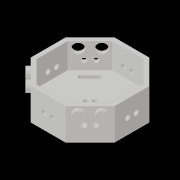
# Autodesk Inventor part: oktagonOben_v2
Saved by Autodesk Inventor 2018.2 (Build 222227000, 227)
## iProperties
Created: 2018-08-16
Part Number: oktagonOben_v2
Material: Generisch
Document SubType Name: Modeling
Designer: PRYADUN
Density: 1 g/cm^3
Appearance: Vorgabe
Mass: 6.7855 g
Surface Area: 62.9444 cm^2
Volume: 6.7855 cm^3
Author: PRYADUN
Autodesk Inventor part; units mm, degrees
sketch "Skizze1" plane through (0, 0, 0) normal (0, 0, 1) x (1, 0, 0)
  line L0 (-8.2843, 20) -> (8.2843, 20)
  line L1 (8.2843, 20) -> (20, 8.2843)
  line L2 (20, 8.2843) -> (20, -8.2843)
  line L3 (20, -8.2843) -> (8.2843, -20)
  line L4 (8.2843, -20) -> (-8.2843, -20)
  line L5 (-8.2843, -20) -> (-20, -8.2843)
  line L6 (-20, -8.2843) -> (-20, 8.2843)
  line L7 (-20, 8.2843) -> (-8.2843, 20)
  line L8 (0, -28) -> (0, 28) projected
  line L9 (-28, 0) -> (28, 0) projected
  point P0 (0, 0)
  dimension "d0" = 40
  dimension "d1" = 40
  constraints: 16 end point, 2 equal length, 2 horizontal, 1 perpendicular, 1 vertical, 5 other
  measures "d0" distance between parallel lines of L4 L0
  measures "d1" distance between parallel lines of L2 L6
extrude "Extrusion1" add sketch "Skizze1" along normal blind 15
sketch "Skizze2" plane through (0, 0, 15) normal (0, 0, 1) x (1, 0, 0)
  line L0 (8.2843, 20) -> (-8.2843, 20) projected
  line L1 (-8.2843, 20) -> (-20, 8.2843) projected
  line L2 (-20, 8.2843) -> (-20, -8.2843) projected
  line L3 (-20, -8.2843) -> (-8.2843, -20) projected
  line L4 (-8.2843, -20) -> (8.2843, -20) projected
  line L5 (8.2843, -20) -> (20, -8.2843) projected
  line L6 (20, -8.2843) -> (20, 8.2843) projected
  line L7 (20, 8.2843) -> (8.2843, 20) projected
  line L8 (-7.4558, 18) -> (7.4558, 18)
  line L9 (7.4558, 18) -> (18, 7.4558)
  line L10 (18, 7.4558) -> (18, -7.4558)
  line L11 (18, -7.4558) -> (7.4558, -18)
  line L12 (7.4558, -18) -> (-7.4558, -18)
  line L13 (-7.4558, -18) -> (-18, -7.4558)
  line L14 (-18, -7.4558) -> (-18, 7.4558)
  line L15 (-18, 7.4558) -> (-7.4558, 18)
  point P0 (0, 0)
  dimension "d4" = 2
  constraints: 16 end point, 7 other
  measures "d4" distance between parallel lines of L0 L8
extrude "Extrusion2" cut sketch "Skizze2" against normal blind 12 contours L8 L9 L10 L11 L12 L13 L14 L15
sketch "Skizze3" plane through (-18, -7.4558, 15) normal (1, 0, 0) x (0, 0, -1)
  line L0 (0, 0) -> (0, 14.9117) projected
  line L1 (0, 0) -> (12, 0) projected
  line L2 (12, 0) -> (12, 14.9117) projected
  line L3 (0, 14.9117) -> (12, 14.9117) projected
  line L4 (12, 0) -> (12, 14.9117) projected
  line L5 (12, 7.4558) -> (0, 7.4558)
  line L6 (0, 0) -> (0, 14.9117) projected
  point P0 (15, 7.4558)
  point P1 (8, 9.4558)
  point P2 (8, 5.4558)
  dimension "d7" = 4
  dimension "d23" = 4
  constraints: 2 end point, 2 midpoint, 1 symmetric about line, 1 vertical alignment
  measures "d7" distance of point (8, 5.456) point (8, 9.456)
  measures "d23" distance from line of L2 point (8, 9.456)
hole "Bohrung1" at (-18, 2, 7) at (-18, -2, 7) direction (-1, 0, 0) diameter 2.2 end through all
mirror "Spiegeln1" about plane through (0, 0, 0) normal (1, 0, 0) of "Bohrung1"
ref_plane "Arbeitsebene1" through (-5.2721, -5.2721, 15) normal (0.7071, -0.7071, 0) x (-0.7071, -0.7071, 0)
mirror "Spiegeln2" about plane through (-5.2721, -5.2721, 15) normal (0.7071, -0.7071, 0) of "Bohrung1"
sketch "Skizze4" plane through (-7.4558, -18, 3) normal (0.7071, 0.7071, 0) x (-0.7071, 0.7071, 0)
  point P0 (7.4558, -3)
ref_plane "Arbeitsebene2" through (-18, -7.4558, 15) normal (0.3827, -0.9239, 0) x (0, 0, -1)
mirror "Spiegeln3" about plane through (-18, -7.4558, 15) normal (0.3827, -0.9239, 0) of "Bohrung1"
mirror "Spiegeln4" about plane through (0, 0, 0) normal (0, 1, 0) of "Bohrung1", "Spiegeln2"
mirror "Spiegeln5" about plane through (0, 0, 0) normal (1, 0, 0) of "Bohrung1", "Spiegeln3"
mirror "Spiegeln6" about plane through (0, 0, 0) normal (0, 1, 0) of "Bohrung1", "Spiegeln3", "Spiegeln5"
sketch "Skizze6" plane through (-8.2843, -20, 15) normal (-0.7071, -0.7071, 0) x (-0.7071, 0.7071, 0)
  circle A0 centre (4.2843, 3.0841) radius 2.3005
  circle A1 centre (6.2843, 8) radius 1.1 projected
  circle A2 centre (10.2843, 8) radius 1.1 projected
  line L0 (0, 15) -> (16.5685, 15) projected
  line L1 (0, 15) -> (0, 0) projected
  line L2 (16.5685, 0) -> (0, 0) projected
  line L3 (16.5685, 15) -> (16.5685, 0) projected
  circle A3 centre (12.2843, 3.0841) radius 2.3005
  line L4 (8.2843, 15) -> (8.2843, 0)
  line L5 (16.5685, 0) -> (0, 0) projected
  dimension "d24" = 4.601
  dimension "d25" = 4.601
  dimension "d26" = 8
  constraints: 2 centre point, 2 end point, 1 horizontal alignment, 1 midpoint, 1 symmetric about line
  measures "d24" diameter of A0
  measures "d25" diameter of A3
  measures "d26" distance of A3.centre A0.centre
extrude "Extrusion3" add sketch "Skizze6" along normal blind 1.8 contours A0 | A3
chamfer "Fase1" distance 0.135 angle 45 2 edges at (-10.9598, -19.8701, 11.9159) (-16.6167, -14.2132, 11.9159)
sketch "Skizze7" plane through (8.2843, 20, 0) normal (0.7071, 0.7071, 0) x (-0.7071, 0.7071, 0)
  circle A0 centre (-4.2843, 11.9159) radius 2.3005 projected
  circle A1 centre (-12.2843, 11.9159) radius 2.3005 projected
  circle A2 centre (-4.2843, 11.9159) radius 2.3985
  circle A3 centre (-12.2843, 11.9159) radius 2.3985
  point P0 (-8.2843, 0)
  dimension "d33" = 4.797
  dimension "d34" = 4.797
  constraints: 2 centre point, 2 coincident
  measures "d33" diameter of A2
  measures "d34" diameter of A3
extrude "Extrusion4" cut sketch "Skizze7" against normal blind 2.2 contours A0 | A1 | A2 | A3
sketch "Skizze8" plane through (0, 0, 0) normal (0, 0, -1) x (-1, 0, 0)
  line L0 (8.2843, 20) -> (-8.2843, 20) projected
  line L1 (-8.2843, 20) -> (-20, 8.2843) projected
  line L2 (-20, 8.2843) -> (-20, -8.2843) projected
  line L3 (-20, -8.2843) -> (-8.2843, -20) projected
  line L4 (-8.2843, -20) -> (8.2843, -20) projected
  line L5 (8.2843, -20) -> (20, -8.2843) projected
  line L6 (20, -8.2843) -> (20, 8.2843) projected
  line L7 (20, 8.2843) -> (8.2843, 20) projected
  line L8 (8.2843, -20) -> (20, -8.2843) projected
  line L9 (14.1421, -14.1421) -> (-14.1421, 14.1421)
  line L10 (-20, 8.2843) -> (-8.2843, 20) projected
  point P0 (0, 0)
  point P1 (1.0607, -1.0607)
  point P2 (-1.0607, 1.0607)
  dimension "d43" = 3
  dimension "d44" = 1.5
  constraints: 2 end point, 2 midpoint, 2 point on line
  measures "d43" distance of point (-1.061, 1.061) point (1.061, -1.061)
  measures "d44" distance of point (0, 0) point (1.061, -1.061)
hole "Bohrung3" at (-1.0607, -1.0607, 0) at (1.0607, 1.0607, 0) direction (0, 0, 1) diameter 1.8 end through all
ref_plane "Arbeitsebene3" through (0, -18, 15) normal (1, 0, 0) x (0, 1, 0)
mirror "Spiegeln7" about plane through (0, -18, 15) normal (1, 0, 0) of "Extrusion3", "Extrusion4"
sketch "Skizze9" plane through (0, 0, 0) normal (0, 0, -1) x (-1, 0, 0)
  circle A0 centre (1.0607, -1.0607) radius 0.9 projected
  circle A1 centre (-1.0607, 1.0607) radius 0.9 projected
  line L0 (8.2843, 20) -> (-8.2843, 20) projected
  line L1 (-8.2843, 20) -> (-20, 8.2843) projected
  line L2 (-20, 8.2843) -> (-20, -8.2843) projected
  line L3 (-20, -8.2843) -> (-8.2843, -20) projected
  line L4 (-8.2843, -20) -> (8.2843, -20) projected
  line L5 (8.2843, -20) -> (20, -8.2843) projected
  line L6 (20, -8.2843) -> (20, 8.2843) projected
  line L7 (20, 8.2843) -> (8.2843, 20) projected
  line L8 (7.0004, 12.7986) -> (7.0004, 12.7986)
  line L9 (7.0004, 11.243) -> (11.243, 7.0004)
  line L10 (12.7986, 7.0004) -> (12.7986, 7.0004)
  line L11 (12.7986, 8.556) -> (8.556, 12.7986)
  line L12 (20, 8.2843) -> (8.2843, 20) projected
  line L13 (0, 0) -> (14.1421, 14.1421)
  arc A2 (11.243, 7.0004) -> (12.7986, 7.0004) centre (12.0208, 7.7782) ccw
  arc A3 (12.7986, 7.0004) -> (12.7986, 8.556) centre (12.0208, 7.7782) ccw
  arc A4 (7.0004, 12.7986) -> (7.0004, 11.243) centre (7.7782, 12.0208) ccw
  arc A5 (8.556, 12.7986) -> (7.0004, 12.7986) centre (7.7782, 12.0208) ccw
  dimension "d52" = 1.1
  dimension "d53" = 1.1
  dimension "d54" = 2.2
  dimension "d55" = 3
  dimension "d58" = 6
  constraints: 10 end point, 8 point on circle, 8 tangent, 4 centre point, 3 parallel, 2 equal radius, 1 midpoint, 1 perpendicular, 1 other
  measures "d52" radius of A2
  measures "d53" radius of A3
  measures "d54" distance between parallel lines of L11 L9
  measures "d55" distance from line of L13 A3.centre
  measures "d58" distance from line of A3.centre L7
extrude "Extrusion5" cut sketch "Skizze9" along normal mid plane 10 contours L11 A3 A2 L9 L13 | L13 L9 A4 A5 L11
equation "\"d1\" = d0"
equation "\"d34\" = d33"
